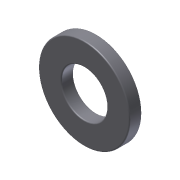
# Autodesk Inventor part: 375 washer structural 112 thick
Saved by Autodesk Inventor 2011 SP1 (Build 150282100, 282)
## iProperties
Created: 2011-07-25
Part Number: 375 washer structural 112 thick
Material: Steel
Document SubType Name: Modeling
Designer: Dan Niemitalo
Mass: 5.47462 g
Surface Area: 7.51505 cm^2
Volume: 0.697404 cm^3
Density: 7.85 g/cm^3
Author: Dan Niemitalo
Autodesk Inventor part; units mm, degrees
ref_plane "YZ Plane" through (0, 0, 0) normal (1, 0, 0) x (0, 1, 0)
ref_plane "XZ Plane" through (0, 0, 0) normal (0, 1, 0) x (-1, 0, 0)
ref_plane "XY Plane" through (0, 0, 0) normal (0, 0, 1) x (1, 0, 0)
sketch "Sketch1" plane through (0, 0, 0) normal (0, 0, 1) x (1, 0, 0)
  circle A0 centre (0, 0) radius 5.1562
  circle A1 centre (0, 0) radius 10.3124
  dimension "d0" = 10.3124
  dimension "d1" = 20.6248
  constraints: 2 centre point, 2 coincident
  measures "d0" diameter of A0
  measures "d1" diameter of A1
extrude "Extrusion1" add sketch "Sketch1" along normal blind 2.794
fillet "Fillet1" radius 0.254 2 edges at (-10.3124, 0, 2.794) (-10.3124, 0, 0)
fillet "Fillet2" radius 0.254 2 edges at (-5.1562, 0, 2.794) (-5.1562, 0, 0)
body "Solid1"
